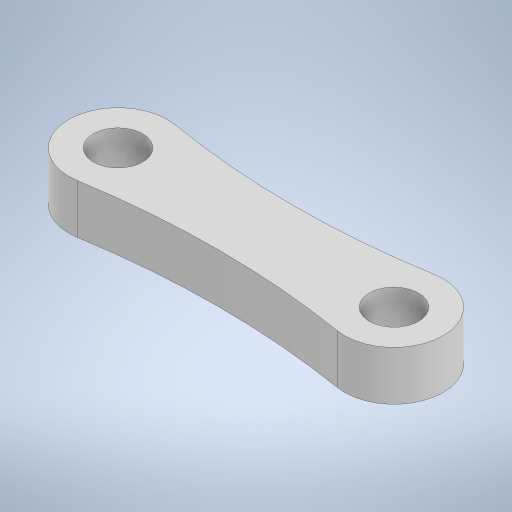
# Autodesk Inventor part: body-connector
Saved by Autodesk Inventor 2024 (Build 280153000, 153)
## iProperties
Created: 2023-10-17
Part Number: body-connector
Material: Generic
Document SubType Name: Modeling
Designer: Piter
Density: 1 g/cm^3
Appearance: Default
Author: Piter
Autodesk Inventor part; units mm, degrees
ref_plane "YZ Plane" through (0, 0, 0) normal (1, 0, 0) x (0, 1, 0)
ref_plane "XZ Plane" through (0, 0, 0) normal (0, 1, 0) x (-1, 0, 0)
ref_plane "XY Plane" through (0, 0, 0) normal (0, 0, 1) x (1, 0, 0)
sketch "Sketch1" plane through (0, 0, 0) normal (0, 1, 0) x (-1, 0, 0)
  line L0 (-22.9214, -0.0293) -> (5.0786, -0.0293)
  circle A0 centre (5.0786, -0.0293) radius 2.5
  circle A1 centre (-22.9214, -0.0293) radius 2.5
  circle A2 centre (-22.9214, -0.0293) radius 5
  circle A3 centre (5.0786, -0.0293) radius 5
  line L1 (-8.9214, -0.0293) -> (-8.9214, -3.8509)
  line L2 (-8.9214, -3.8509) -> (-8.9214, -0.0293)
  line L3 (-8.9214, -0.0293) -> (-8.9214, 3.8269)
  arc A4 (-22.1098, 4.9044) -> (4.267, 4.9044) centre (-8.9214, 85.0769) ccw
  arc A5 (4.2428, -4.9589) -> (-22.0856, -4.9589) centre (-8.9214, -82.6063) ccw
  point P0 (0, 0)
  dimension "d0" = 28
  dimension "d1" = 5
  dimension "d2" = 5
  dimension "d3" = 10
  dimension "d4" = 10
  constraints: 10 point on circle, 8 end point, 6 centre point, 4 coincident, 4 tangent, 2 vertical, 1 collinear, 1 horizontal, 1 midpoint
  measures "d0" distance of L0.start L0.end
  measures "d1" diameter of A0
  measures "d2" diameter of A1
  measures "d3" diameter of A2
  measures "d4" diameter of A3
extrude "Extrusion1" add sketch "Sketch1" along normal blind 5
body "Solid1"
